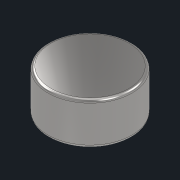
# Autodesk Inventor part: holder_magnet
Saved by Autodesk Inventor 2021 (Build 250183000, 183)
## iProperties
Created: 2020-09-05
Part Number: holder_magnet
Material: 鋼、炭素鋼
Document SubType Name: Modeling
Designer: Yuta Kage
Mass: 0.441405 g
Surface Area: 0.909761 cm^2
Volume: 0.0562299 cm^3
Density: 7.85 g/cm^3
Appearance: 半つや出し
Description: 購入済
Author: Yuta Kage
Autodesk Inventor part; units mm, degrees
ref_plane "YZ Plane" through (0, 0, 0) normal (1, 0, 0) x (0, 1, 0)
ref_plane "XZ Plane" through (0, 0, 0) normal (0, 1, 0) x (-1, 0, 0)
ref_plane "XY Plane" through (0, 0, 0) normal (0, 0, 1) x (1, 0, 0)
sketch "スケッチ1" plane through (0, 0, 0) normal (0, 1, 0) x (-1, 0, 0)
  circle A0 centre (0, 0) radius 3
  dimension "d0" = 6
  constraints: 1 centre point, 1 coincident
  measures "d0" diameter of A0
extrude "押し出し1" add sketch "スケッチ1" along normal blind 3
fillet "フィレット1" radius 0.2 2 edges at (3, 3, 0) (3, 0, 0)
